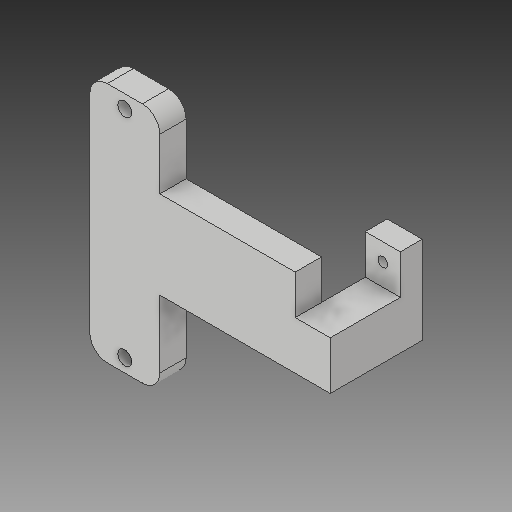
# Autodesk Inventor part: HbServoCover
Saved by Autodesk Inventor 2017.3 (Build 213256000, 256)
## iProperties
Part Number: HbServoCover
Material: 一般
Document SubType Name: Modeling
Designer: sktom
Density: 1 g/cm^3
Appearance: 既定
Author: sktom
Autodesk Inventor part; units mm, degrees
ref_plane "YZ Plane" through (0, 0, 0) normal (1, 0, 0) x (0, 1, 0)
ref_plane "XZ Plane" through (0, 0, 0) normal (0, 1, 0) x (-1, 0, 0)
ref_plane "XY Plane" through (0, 0, 0) normal (0, 0, 1) x (1, 0, 0)
sketch "スケッチ1" plane through (0, 0, 0) normal (0, 0, 1) x (1, 0, 0)
  circle A0 centre (0, 12.3) radius 0.8
  circle A1 centre (0, -12.3) radius 0.8
  line L0 (-4, -13.8) -> (4, -13.8)
  line L1 (4, -13.8) -> (4, 13.8)
  line L2 (4, 13.8) -> (-4, 13.8)
  line L3 (-4, 13.8) -> (-4, -13.8)
  line L4 (-4, -13.8) -> (4, 13.8) construction
  line L5 (4, -13.8) -> (-4, 13.8) construction
  point P0 (0, 0)
  dimension "d0" = 1.6
  dimension "d1" = 24.6
  dimension "d2" = 12.3
  dimension "d3" = 1.5
  dimension "d4" = 4
  constraints: 12 end point, 2 centre point, 2 midpoint, 2 parallel, 2 vertical alignment, 1 equal radius, 1 horizontal, 1 perpendicular
  measures "d0" diameter of A0
  measures "d1" distance of A1.centre A0.centre
  measures "d2" distance of point (0, 0) A1.centre
  measures "d3" distance from line of A0.centre L2
  measures "d4" distance from line of A0.centre L3
extrude "押し出し1" add sketch "スケッチ1" along normal blind 3
sketch "スケッチ2" plane through (0, 0, 3) normal (0, 0, 1) x (1, 0, 0)
  circle A0 centre (21.45, 3.898) radius 0.55 projected
  line L0 (19.45, 5.898) -> (19.45, -4.102) projected
  line L1 (19.45, -4.102) -> (23.45, -4.102) projected
  line L2 (23.45, -4.102) -> (23.45, 5.898) projected
  line L3 (23.45, 5.898) -> (19.45, 5.898) projected
  line L4 (23.45, -4.102) -> (4, -4.102)
  line L5 (4, -4.102) -> (4, 5.898)
  line L6 (4, 5.898) -> (23.45, 5.898)
  line L7 (23.45, 5.898) -> (23.45, -4.102)
  line L8 (4, -13.8) -> (4, 13.8) projected
  point P0 (0, 0)
  constraints: 8 end point, 2 parallel, 1 collinear, 1 horizontal, 1 perpendicular, 1 point on line
extrude "押し出し2" add sketch "スケッチ2" against normal up to surface (3 mm away)
sketch "スケッチ3" plane through (0, 0, 0) normal (0, 0, -1) x (-1, 0, 0)
  circle A0 centre (-21.45, 3.898) radius 0.55 projected
  line L0 (-19.45, 5.898) -> (-19.45, -4.102) projected
  line L1 (-19.45, -4.102) -> (-23.45, -4.102) projected
  line L2 (-23.45, -4.102) -> (-23.45, 5.898) projected
  line L3 (-23.45, 5.898) -> (-19.45, 5.898) projected
  point P0 (0, 0)
ref_plane "作業平面1" through (19.45, -4.102, -7.5) normal (0, 0, 1) x (1, 0, 0)
extrude "押し出し3" add sketch "スケッチ3" along normal up to surface (7.5 mm away)
sketch "スケッチ4" plane through (0, 0, 3) normal (0, 0, 1) x (1, 0, 0)
  line L0 (23.45, -4.102) -> (23.45, 5.898) projected
  line L1 (19.45, 5.898) -> (19.45, -4.102) projected
  line L2 (23.45, 5.898) -> (19.45, 5.898)
  line L3 (19.45, 5.898) -> (19.45, 1.398)
  line L4 (19.45, 1.398) -> (23.45, 1.398)
  line L5 (23.45, 1.398) -> (23.45, 5.898)
  point P0 (0, 0)
  dimension "d11" = 4.5
  constraints: 8 end point, 2 parallel, 1 horizontal, 1 perpendicular, 1 point on line
  measures "d11" distance between parallel lines of L2 L4
extrude "押し出し4" cut sketch "スケッチ4" against normal blind 8
fillet "フィレット1" radius 2 4 edges at (4, -13.8, 1.5) (-4, -13.8, 1.5) (4, 13.8, 1.5) (-4, 13.8, 1.5)
